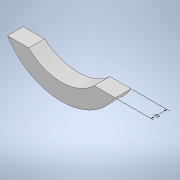
# Autodesk Inventor part: electricLightCover
Saved by Autodesk Inventor 2020.3 (Build 243373000, 373)
## iProperties
Created: 2020-05-22
Part Number: electricLightCover
Material: Generic
Document SubType Name: Modeling
Designer: robst
Density: 1 g/cm^3
Appearance: Default
Author: robst
Autodesk Inventor part; units mm, degrees
ref_plane "YZ Plane" through (0, 0, 0) normal (1, 0, 0) x (0, 1, 0)
ref_plane "XZ Plane" through (0, 0, 0) normal (0, 1, 0) x (-1, 0, 0)
sketch "Sketch1" plane through (0, 0, 0) normal (0, 0, 1) x (1, 0, 0)
  arc A0 (-51.2937, -31.75) -> (51.2937, -31.75) centre (0, 0) ccw
  arc A1 (-31.1085, -31.75) -> (31.1085, -31.75) centre (0, 0) ccw
  line L0 (-50.8, 0) -> (50.8, 0) construction
  line L1 (-51.2937, -31.75) -> (51.2937, -31.75)
  dimension "outerDiameter" = 120.65
  dimension "innerDiameter" = 88.9
  dimension "distanceBelowCenterLine" = 31.75
  constraints: 4 end point, 4 point on circle, 2 centre point, 2 coincident, 2 horizontal, 2 point on line
  measures "outerDiameter" diameter of A0
  measures "innerDiameter" diameter of A1
  measures "distanceBelowCenterLine" distance from line of L1 point (0, 0)
ref_plane "Work Plane3" through (-50.8, 1.0626, -12.1456) normal (0, -0.0871557, 0.9961947) x (1, 0, 0)
ref_plane "Work Plane2" through (-50.8, 0, 0) normal (0, -0.0871557, 0.9961947) x (1, 0, 0)
extrude "Extrusion1" add sketch "Sketch1" against normal up to surface contours L1 A1 A0 surface through (-50.8, 1.0626, -12.1456) normal (0, -0.0871557, 0.9961947)
body "Solid1"
